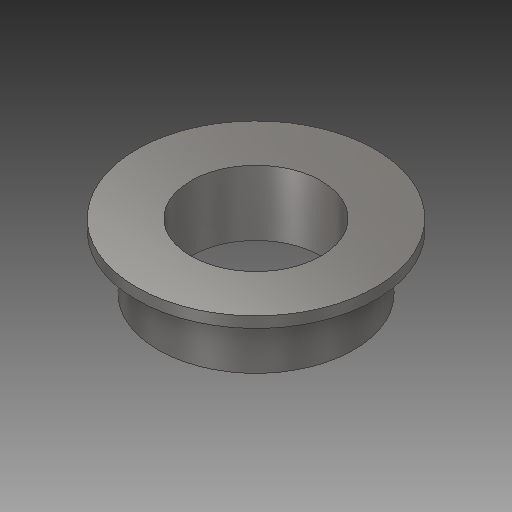
# Autodesk Inventor part: bearing_outer
Saved by Autodesk Inventor 2017 (Build 210142000, 142)
## iProperties
Created: 2017-01-16
Part Number: bearing_outer
Material: Steel, Alloy
Document SubType Name: Modeling
Designer: mmarkle
Density: 7.73 g/cm^3
Appearance: Semi-Polished
Mass: 30.1184 g
Surface Area: 28.0273 cm^2
Volume: 3.8963 cm^3
Author: mmarkle
Autodesk Inventor part; units mm, degrees
ref_plane "YZ Plane" through (0, 0, 0) normal (1, 0, 0) x (0, 1, 0)
ref_plane "XZ Plane" through (0, 0, 0) normal (0, 1, 0) x (-1, 0, 0)
ref_plane "XY Plane" through (0, 0, 0) normal (0, 0, 1) x (1, 0, 0)
sketch "Sketch1" plane through (0, 0, 0) normal (1, 0, 0) x (0, 1, 0)
  line L0 (10.6665, 0) -> (-4.583, 0)
  line L1 (0, 0) -> (0, 14.2875)
  line L2 (0, 14.2875) -> (7.9375, 14.2875)
  line L3 (7.9375, 14.2875) -> (7.9375, 17.4625)
  line L4 (7.9375, 17.4625) -> (9.525, 17.4625)
  line L5 (9.525, 17.4625) -> (9.525, 0)
  line L6 (9.525, 0) -> (0, 0)
  dimension "d2" = 3.175
  dimension "d3" = 1.5875
  dimension "d4" = 28.575
  dimension "d5" = 9.525
  constraints: 14 end point, 4 perpendicular, 1 collinear, 1 horizontal, 1 point on line, 1 vertical
  measures "d2" distance of L2.end L3.end
  measures "d3" distance of L3.end L4.end
  measures "d4" diameter of L1.end L0
  measures "d5" distance between parallel lines of L1 L5
revolve "Revolution1" add sketch "Sketch1" angle 360 about axis through (0, 10.6665, 0) along (0, -1, 0)
sketch "Sketch2" plane through (0, 9.525, 0) normal (0, 1, 0) x (1, 0, 0)
  circle A0 centre (0, 0) radius 9.525
  dimension "d7" = 19.05
  constraints: 1 centre point, 1 coincident
  measures "d7" diameter of A0
extrude "Extrusion1" cut sketch "Sketch2" against normal blind 25.4
body "Solid1"
